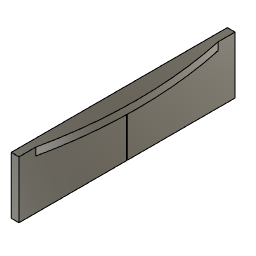
Bridge Radius Line Jig - 14 Inch (Autodesk Fusion 360 design; units mm, degrees)
Autodesk Fusion 360 part; units mm, degrees
sketch "Sketch1" plane through (0, 0, 0) normal (0, 0, 1) x (1, 0, 0)
  circle A0 centre (0, 0) radius 355.6
  line L0 (444.5, 203.2) -> (436.499, 203.2)
  line L1 (436.499, 203.2) -> (436.499, 12.7)
  line L2 (436.499, 12.7) -> (444.5, 12.7)
  line L3 (444.5, 12.7) -> (444.5, 203.2)
  line L4 (355.6, 0.0349) -> (347.599, 0.0349)
  line L5 (347.599, 0.0349) -> (341.249, 0.0349)
  line L6 (341.249, 0.0349) -> (341.249, -88.8651)
  line L7 (341.249, -88.8651) -> (347.599, -88.8651)
  line L8 (347.599, -88.8651) -> (347.599, 0.0349)
  line L9 (347.599, 0.0349) -> (341.249, 0.0349)
  line L10 (341.249, 0.0349) -> (341.249, 88.9349)
  line L11 (341.249, 88.9349) -> (347.599, 88.9349)
  line L12 (347.599, 88.9349) -> (347.599, 0.0349)
  dimension "d1" = 711.2
  dimension "d2" = 8.001
  dimension "d3" = 190.5
  dimension "d4" = 8.001
  dimension "d5" = 6.35
  dimension "d6" = 88.9
  dimension "d7" = 6.35
  dimension "d8" = 88.9
  constraint coincident A0.centre origin
  constraint horizontal L0
  constraint vertical L1
  constraint horizontal L2
  constraint vertical L3
  constraint coincident A0 L4.start
  constraint horizontal L4
  constraint horizontal L5
  constraint vertical L6
  constraint horizontal L7
  constraint vertical L8
  constraint horizontal L9
  constraint vertical L10
  constraint horizontal L11
  constraint vertical L12
  measures "d1" diameter of A0
  measures "d2" distance of L0.start L0.end
  measures "d3" distance of L0.start L2.end
  measures "d4" distance of L4.start L4.end
  measures "d5" distance of L4.end L5.end
  measures "d6" distance of L4.end L7.end
  measures "d7" distance of L4.end L5.end
  measures "d8" distance of L4.end L11.end
extrude "Extrude1" add sketch "Sketch1" along normal blind 6.35 contours A0 L4 L8 | A0 L4 L12 | A0 L7 L8 | A0 L5 L6 L7 L8 L9 | A0 L5 L9 L10 L11 L12 | A0 L11 L12
sketch "Sketch2" plane through (0, 0, 0) normal (0, 0, -1) x (1, 0, 0)
  line L0 (341.249, 88.8651) -> (341.249, -88.9349)
  line L1 (341.249, -88.9349) -> (347.599, -88.9349)
  line L2 (347.599, -88.9349) -> (347.599, -75.0086)
  arc A0 (347.599, -75.0086) -> (347.599, 75.0086) centre (0, 0) ccw
  line L3 (347.599, 75.0086) -> (347.599, 88.8651)
  line L4 (347.599, 88.8651) -> (341.249, 88.8651)
  line L5 (341.249, 88.8651) -> (347.599, 88.8651)
  line L6 (347.599, 88.8651) -> (347.599, -88.9349)
  line L7 (347.599, -88.9349) -> (341.249, -88.9349)
  line L8 (341.249, -88.9349) -> (341.249, 88.8651)
  constraint horizontal L5
  constraint vertical L6
  constraint horizontal L7
  constraint vertical L8
  constraint coincident L1.end L2.start
  constraint coincident L0.start L4.end
extrude "Extrude2" add sketch "Sketch2" along normal blind 40.64 contours L0 L1 L2 L3 L4 L5 L6 L7 L8
sketch "Sketch3" plane through (347.599, 0, 0) normal (1, 0, 0) x (0, 1, 0)
  line L0 (-75.0086, 0) -> (-75.0086, 6.35)
  line L1 (-75.0086, 6.35) -> (-88.8651, 6.35)
  line L2 (-88.8651, 6.35) -> (-88.8651, -40.64)
  line L3 (-88.8651, -40.64) -> (88.9349, -40.64)
  line L4 (88.9349, -40.64) -> (88.9349, 6.35)
  line L5 (88.9349, 6.35) -> (75.0086, 6.35)
  line L6 (75.0086, 6.35) -> (75.0086, 0)
  line L7 (75.0086, 0) -> (-75.0086, 0)
  line L8 (0.0349, -40.64) -> (-0.1842, -40.64)
  line L9 (-0.1842, -40.64) -> (-0.1842, 0)
  line L10 (-0.1842, 0) -> (0.0349, 0)
  line L11 (0.0349, 0) -> (0.0349, -40.64)
  line L12 (0.254, 0) -> (0.0349, 0)
  line L13 (0.0349, 0) -> (0.0349, -40.64)
  line L14 (0.0349, -40.64) -> (0.254, -40.64)
  line L15 (0.254, -40.64) -> (0.254, 0)
  constraint horizontal L8
  constraint vertical L9
  constraint horizontal L10
  constraint vertical L11
  constraint coincident L7 L9.end
  constraint midpoint L3 L8.start
  constraint horizontal L12
  constraint vertical L13
  constraint horizontal L14
  constraint vertical L15
  constraint coincident L7 L12.start
  constraint symmetric L9 L11 L15
emboss "Emboss1" depth -0.254 profiles "Sketch3" section 1 contours L3 L7 L8 L9 L10 L11 L13 | L3 L7 L11 L12 L13 L14 L15 onto face at (347.599, 25.0262, -27.0933)
